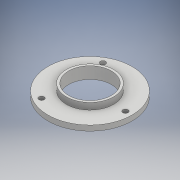
# Autodesk Inventor part: ACO.RODA15-02
Saved by Autodesk Inventor 2018 (Build 220112000, 112)
## iProperties
Created: 2018-02-28
Part Number: ACO.RODA15-02
Material: Generic
Document SubType Name: Modeling
Designer: isai
Density: 1 g/cm^3
Appearance: Default
Author: isai
Autodesk Inventor part; units mm, degrees
ref_plane "YZ Plane" through (0, 0, 0) normal (1, 0, 0) x (0, 1, 0)
ref_plane "XZ Plane" through (0, 0, 0) normal (0, 1, 0) x (-1, 0, 0)
ref_plane "XY Plane" through (0, 0, 0) normal (0, 0, 1) x (1, 0, 0)
sketch "Sketch1" plane through (0, 0, 0) normal (0, 0, 1) x (1, 0, 0)
  circle A0 centre (0, 0) radius 16.25
  circle A1 centre (0, 0) radius 18
  circle A2 centre (0, 0) radius 32
  dimension "d0" = 32.5
  dimension "d16" = 64
  dimension "d21" = 36
  constraints: 3 centre point, 1 coincident
  measures "d0" diameter of A0
  measures "d16" diameter of A2
  measures "d21" diameter of A1
extrude "Extrusion1" add sketch "Sketch1" along normal blind 4 contours A2
extrude "Extrusion2" add sketch "Sketch1" along normal blind 9 contours A1
sketch "Sketch2" plane through (0, 0, 4) normal (0, 0, 1) x (1, 0, 0)
  circle A0 centre (0, 0) radius 32 projected
  circle A1 centre (27, 0) radius 2
  circle A2 centre (-13.5, 23.3827) radius 2
  circle A3 centre (-13.5, -23.3827) radius 2
  dimension "d8" = 4
  dimension "d9" = 27
  dimension "d12" = 360
  constraints: 3 centre point, 7 other
  measures "d8" diameter of A1
  measures "d9" distance of point (0, 0) A1.centre
extrude "Extrusion3" cut sketch "Sketch2" against normal up to surface (4 mm away) contours A1 | A2 | A3
equation "\"d0\" = a"
equation "\"a\" = 32.5"
body "Solid1"
